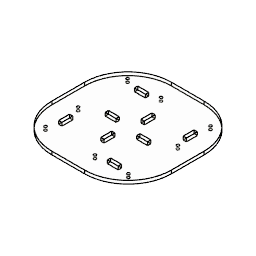
BasePlate_v7 (Autodesk Fusion 360 design; units mm, degrees)
Autodesk Fusion 360 part; units mm, degrees
sketch "Sketch1" plane through (0, 0, 0) normal (0, 0, 1) x (1, 0, 0)
  line L0 (-33.4, -17.4) -> (-33.4, 33.4) construction
  line L1 (-33.4, 33.4) -> (-27.4, 33.4) construction
  line L2 (-33.4, -17.4) -> (-36.4, -17.4)
  line L3 (-36.4, -17.4) -> (-36.4, -27.4)
  line L4 (-36.4, -27.4) -> (-33.4, -27.4)
  line L5 (-33.4, -27.4) -> (-33.4, -17.4)
  line L6 (-27.4, 33.4) -> (-17.4, 33.4)
  line L7 (-17.4, 33.4) -> (-17.4, 36.4)
  line L8 (-17.4, 36.4) -> (-27.4, 36.4)
  line L9 (-27.4, 36.4) -> (-27.4, 33.4)
  line L10 (-17.4, 33.4) -> (33.4, 33.4) construction
  line L11 (33.4, 33.4) -> (33.4, 27.4) construction
  line L12 (33.4, 27.4) -> (36.4, 27.4)
  line L13 (36.4, 27.4) -> (36.4, 17.4)
  line L14 (36.4, 17.4) -> (33.4, 17.4)
  line L15 (33.4, 17.4) -> (33.4, 27.4)
  line L16 (33.4, 17.4) -> (33.4, -33.4) construction
  line L17 (33.4, -33.4) -> (27.4, -33.4) construction
  line L18 (27.4, -33.4) -> (17.4, -33.4)
  line L19 (17.4, -33.4) -> (17.4, -36.4)
  line L20 (17.4, -36.4) -> (27.4, -36.4)
  line L21 (27.4, -36.4) -> (27.4, -33.4)
  line L22 (17.4, -33.4) -> (-33.4, -33.4) construction
  line L23 (-33.4, -33.4) -> (-33.4, -27.4) construction
  line L24 (33.4, 33.4) -> (-33.4, -33.4) construction
  line L25 (33.4, -33.4) -> (-33.4, 33.4) construction
  line L26 (55, -55) -> (-55, -55)
  line L27 (-55, -55) -> (-55, 55)
  line L28 (-55, 55) -> (55, 55)
  line L29 (55, 55) -> (55, -55)
  line L30 (55, -55) -> (-55, 55) construction
  line L31 (-55, -55) -> (55, 55) construction
  line L32 (-34.9, -17.4) -> (-34.9, -7.75) construction
  line L33 (-34.9, -7.75) -> (-38.15, -7.75) construction
  circle A0 centre (-38.15, -7.75) radius 1.25
  line L34 (-34.9, -27.4) -> (-34.9, -38.15) construction
  line L35 (-34.9, -38.15) -> (-37.75, -38.15) construction
  circle A1 centre (-37.75, -38.15) radius 1.25
  circle A2 centre (38.15, -37.75) radius 1.25
  circle A3 centre (7.75, -38.15) radius 1.25
  circle A4 centre (37.75, 38.15) radius 1.25
  circle A5 centre (38.15, 7.75) radius 1.25
  circle A6 centre (-38.15, 37.75) radius 1.25
  circle A7 centre (-7.75, 38.15) radius 1.25
  line L36 (0, 0) -> (0, 11.5) construction
  line L37 (0, 11.5) -> (3.5, 11.5) construction
  line L38 (3.5, 11.5) -> (0.5, 11.5)
  line L39 (0.5, 11.5) -> (0.5, 21.5)
  line L40 (0.5, 21.5) -> (3.5, 21.5)
  line L41 (3.5, 21.5) -> (3.5, 11.5)
  line L42 (-21.5, 3.5) -> (-11.5, 3.5)
  line L43 (-21.5, 0.5) -> (-21.5, 3.5)
  line L44 (-11.5, 0.5) -> (-21.5, 0.5)
  line L45 (-11.5, 3.5) -> (-11.5, 0.5)
  line L46 (-3.5, -21.5) -> (-3.5, -11.5)
  line L47 (-0.5, -21.5) -> (-3.5, -21.5)
  line L48 (-0.5, -11.5) -> (-0.5, -21.5)
  line L49 (-3.5, -11.5) -> (-0.5, -11.5)
  line L50 (21.5, -3.5) -> (11.5, -3.5)
  line L51 (21.5, -0.5) -> (21.5, -3.5)
  line L52 (11.5, -0.5) -> (21.5, -0.5)
  line L53 (11.5, -3.5) -> (11.5, -0.5)
  dimension "d1" = 50.8
  dimension "d2" = 6
  dimension "d3" = 3
  dimension "d4" = 10
  dimension "d5" = 10
  dimension "d6" = 3
  dimension "d7" = 50.8
  dimension "d8" = 6
  dimension "d9" = 3
  dimension "d10" = 10
  dimension "d11" = 50.8
  dimension "d12" = 6
  dimension "d13" = 10
  dimension "d14" = 3
  dimension "d15" = 50.8
  dimension "d16" = 110
  dimension "d17" = 110
  dimension "d22" = 9.65
  dimension "d23" = 3.25
  dimension "d24" = 2.5
  dimension "d25" = 10.75
  dimension "d26" = 2.85
  dimension "d27" = 2.5
  dimension "d29" = 360
  dimension "d34" = 11.5
  dimension "d36" = 3
  dimension "d37" = 10
  dimension "d39" = 360
  dimension "d40" = 0.5
  constraint vertical L0
  constraint perpendicular L0 L1
  constraint horizontal L2
  constraint vertical L3
  constraint horizontal L4
  constraint vertical L5
  constraint horizontal L6
  constraint vertical L7
  constraint horizontal L8
  constraint vertical L9
  constraint perpendicular L7 L10
  constraint perpendicular L10 L11
  constraint horizontal L12
  constraint vertical L13
  constraint horizontal L14
  constraint vertical L15
  constraint perpendicular L14 L16
  constraint perpendicular L16 L17
  constraint horizontal L18
  constraint vertical L19
  constraint horizontal L20
  constraint vertical L21
  constraint perpendicular L19 L22
  constraint coincident L36.start L24
  constraint coincident L36.start L25
  constraint horizontal L26
  constraint perpendicular L26 L27
  constraint parallel L26 L28
  constraint parallel L27 L29
  constraint coincident L30 L36.start
  constraint coincident L31 L36.start
  constraint coincident L36.start origin
  constraint midpoint L2 L32.start
  constraint perpendicular L2 L32
  constraint perpendicular L32 L33
  constraint coincident L33.end A0.centre
  constraint midpoint L4 L34.start
  constraint perpendicular L4 L34
  constraint perpendicular L34 L35
  constraint coincident L35.end A1.centre
  constraint vertical L36
  constraint horizontal L37
  constraint horizontal L38
  constraint vertical L39
  constraint horizontal L40
  constraint vertical L41
  measures "d1" distance of L0.start L0.end
  measures "d2" distance of L0.end L1.end
  measures "d3" distance of L0.start L2.end
  measures "d4" distance of L0.start L4.end
  measures "d5" distance of L1.end L6.end
  measures "d6" distance of L1.end L8.end
  measures "d7" distance of L6.end L10.end
  measures "d8" distance of L10.end L11.end
  measures "d9" distance of L11.end L12.end
  measures "d10" distance of L11.end L14.end
  measures "d11" distance of L14.end L16.end
  measures "d12" distance of L16.end L17.end
  measures "d13" distance of L17.end L18.end
  measures "d14" distance of L17.end L20.end
  measures "d15" distance of L18.end L22.end
  measures "d16" distance of L27.end L28.end
  measures "d17" distance of L26.end L27.end
  measures "d22" distance of L32.start L32.end
  measures "d23" distance of L32.end L33.end
  measures "d24" diameter of A0
  measures "d25" distance of L34.start L34.end
  measures "d26" distance of L34.end L35.end
  measures "d27" diameter of A1
  measures "d34" distance of L36.start L36.end
  measures "d36" distance of L37.end L38.end
  measures "d37" distance of L37.end L40.end
  measures "d40" distance of L36 L39
extrude "Extrude1" add sketch "Sketch1" along normal blind 3 contours L26 L27 L28 L29 | A0 | A1 | A2 | A3 | A4 | A5 | A6 | A7 | L38 L39 L40 L41 | L42 L43 L44 L45 | L46 L47 L48 L49 | L50 L51 L52 L53
extrude "Extrude2" cut sketch "Sketch1" along normal blind 3 contours A0 | A1 | A2 | A3 | A4 | A5 | A6 | A7 | L38 L39 L40 L41 | L42 L43 L44 L45 | L46 L47 L48 L49 | L50 L51 L52 L53
fillet "Fillet1" radius 40 4 edges at (55, -55, 1.5) (-55, -55, 1.5) (55, 55, 1.5) (-55, 55, 1.5)
